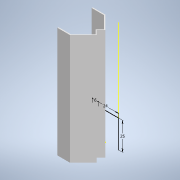
# Autodesk Inventor part: guardv2
Saved by Autodesk Inventor 2022 (Build 260153000, 153)
## iProperties
Created: 2022-06-20
Part Number: guardv2
Material: Generic
Document SubType Name: Modeling
Designer: Cody
Density: 1 g/cm^3
Appearance: Default
Author: Cody
Autodesk Inventor part; units mm, degrees
ref_plane "YZ Plane" through (0, 0, 0) normal (1, 0, 0) x (0, 1, 0)
ref_plane "XZ Plane" through (0, 0, 0) normal (0, 1, 0) x (-1, 0, 0)
ref_plane "XY Plane" through (0, 0, 0) normal (0, 0, 1) x (1, 0, 0)
sketch "Sketch1" plane through (0, 0, 0) normal (0, 1, 0) x (-1, 0, 0)
  line L0 (0, 0) -> (11.2054, 0) construction
  line L1 (11.2054, 0) -> (0, 0) construction
  line L2 (-7.2218, -15) -> (-11.1109, -11.1109) construction
  line L3 (0, 0) -> (-11.1109, -11.1109) construction
  line L4 (-11.1109, -11.1109) -> (-7.2218, -15) construction
  line L5 (-11.1109, -18.8891) -> (0, -30) construction
  line L6 (-7.2218, -15) -> (-11.1109, -18.8891) construction
  line L7 (0, -30) -> (11.2054, -30) construction
  line L8 (11.2054, -30) -> (0, -30) construction
  line L9 (11.2054, -30) -> (11.2054, 0) construction
  line L10 (11.2054, 0) -> (11.2054, -30) construction
  line L11 (11.2054, 0) -> (11.2054, 1)
  line L12 (11.2054, 1) -> (0, 1)
  line L13 (0, 1) -> (-12.1109, -11.1109)
  line L14 (-12.1109, -11.1109) -> (-8.2218, -15)
  line L15 (-8.2218, -15) -> (-12.1109, -18.8891)
  line L16 (-12.1109, -18.8891) -> (0, -31)
  line L17 (0, -31) -> (11.2054, -31)
  line L18 (11.2054, -31) -> (11.2054, -30)
  line L19 (11.2054, -30) -> (0, -30)
  line L20 (-11.1109, -18.8891) -> (0, -30)
  line L21 (-11.1109, -18.8891) -> (-7.2218, -15)
  line L22 (-11.1109, -11.1109) -> (0, 0)
  line L23 (-11.1109, -11.1109) -> (-7.2218, -15)
  line L24 (11.2054, 0) -> (0, 0)
  point P0 (-20.2218, 0)
  dimension "d0" = 1
  constraints: 50 end point, 7 perpendicular, 6 collinear, 4 horizontal, 2 parallel, 1 vertical
  measures "d0" distance of L0.end L11.end
extrude "Extrusion1" add sketch "Sketch1" along normal blind 100
sketch "Sketch3" plane through (-11.2054, 0, 1) normal (0, 0, 1) x (1, 0, 0)
  line L0 (11.2053, -0.0014) -> (11.2053, 99.9986)
  line L1 (11.2053, 99.9986) -> (7.4271, 77.9986)
  circle A0 centre (7.4271, 74.9986) radius 3
  circle A1 centre (7.4271, 74.9986) radius 3
  line L2 (7.4271, 71.9986) -> (7.4271, 27.9986)
  circle A2 centre (7.4271, 24.9986) radius 3
  circle A3 centre (7.4271, 24.9986) radius 3
  point P0 (11.2054, 0)
  point P1 (0, 0)
  constraints: 6 end point, 3 vertical alignment, 2 coincident, 1 centre point, 1 vertical, 7 other
extrude "Extrusion2" cut sketch "Sketch3" against normal up to surface (32 mm away)
body "Solid1"
